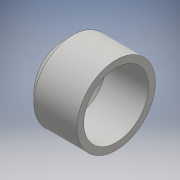
# Autodesk Inventor part: vacum_cap
Saved by Autodesk Inventor 2016 (Build 200138000, 138)
## iProperties
Created: 2016-10-10
Part Number: vacum_cap
Material: Generic
Document SubType Name: Modeling
Designer: rawrdong
Density: 1 g/cm^3
Appearance: Default
Author: rawrdong
Autodesk Inventor part; units mm, degrees
ref_plane "YZ Plane" through (0, 0, 0) normal (1, 0, 0) x (0, 1, 0)
ref_plane "XZ Plane" through (0, 0, 0) normal (0, 1, 0) x (-1, 0, 0)
ref_plane "XY Plane" through (0, 0, 0) normal (0, 0, 1) x (1, 0, 0)
sketch "Sketch1" plane through (0, 0, 0) normal (0, 1, 0) x (-1, 0, 0)
  line L0 (23, 0) -> (23, -17.25)
  line L1 (23, -17.25) -> (0, -17.25)
  line L2 (0, -17.25) -> (0, -14.25)
  line L3 (0, -14.25) -> (20, -13.5516)
  line L4 (20, -13.5516) -> (20, 0)
  line L5 (20, 0) -> (23, 0)
  line L6 (0, 0) -> (20, 0) construction
  dimension "d0" = 2
  dimension "d1" = 28.5
  dimension "d2" = 20
  dimension "d3" = 3
  dimension "d4" = 3
  dimension "d14" = 27.1032
  constraints: 14 end point, 2 horizontal, 2 perpendicular, 2 vertical, 1 vertical alignment
  measures "d0" angle of L1 L3
  measures "d1" diameter of L2.end L6
  measures "d2" distance between parallel lines of L2 L4
  measures "d3" distance between parallel lines of L0 L4
  measures "d4" distance of L1.end L2.end
  measures "d14" diameter of L3.end L6
revolve "Revolution1" add sketch "Sketch1" angle 360 about axis through (0, 0, 0) along (-1, 0, 0)
chamfer "Chamfer1" distance 4 angle 45 1 edges at (-23, 0, 17.25)
chamfer "Chamfer2" distance 2 angle 45 1 edges at (-20, 0, 13.5516)
body "Solid1"
